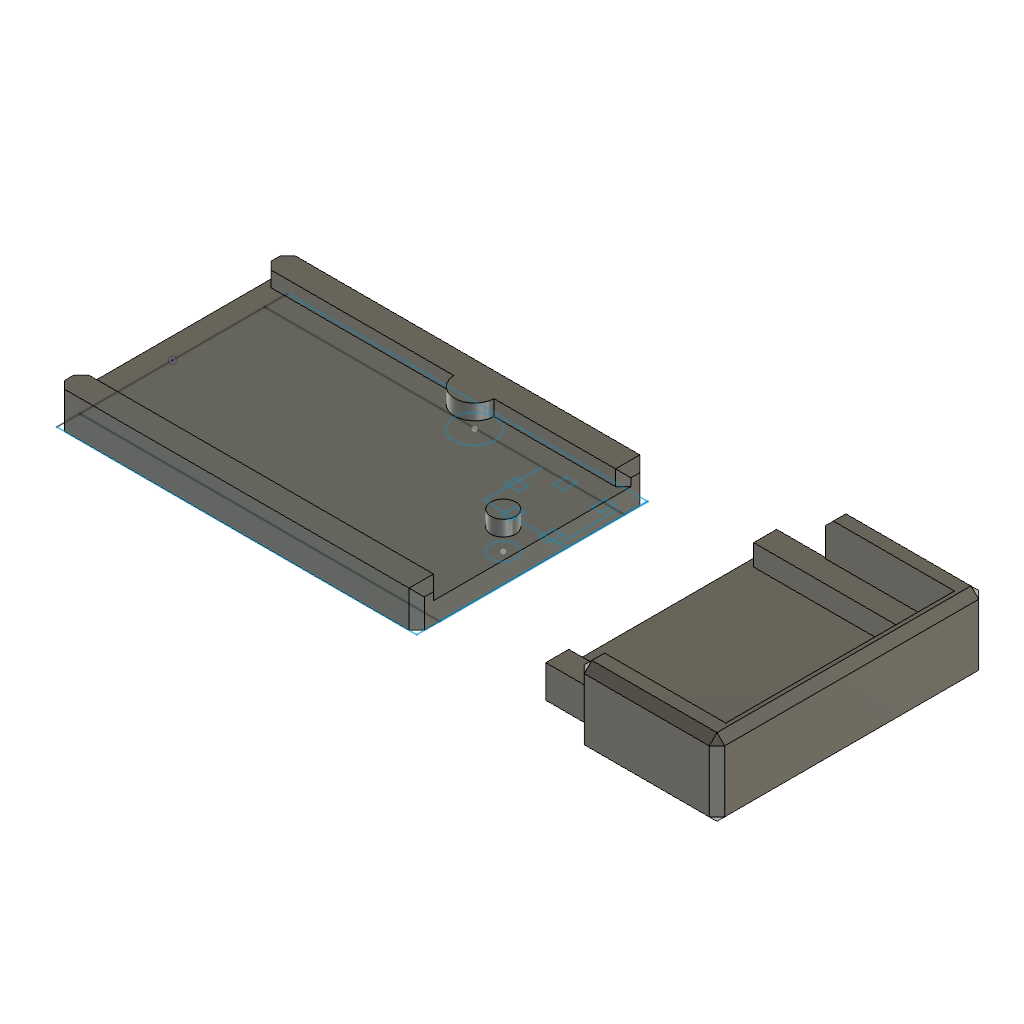
CH552_dongle (Autodesk Fusion 360 design; units mm, degrees)
description: Designed by EasyEDA Pro
part number: EasyEDA PCB Model~ES4X
Autodesk Fusion 360 part; units mm, degrees
sketch "スケッチ1" plane through (0, 0, 0) normal (0, 0, 1) x (1, 0, 0)
  line L0 (0, 4.8) -> (18.7, 4.8)
  line L1 (18.7, -4.8) -> (0, -4.8)
  line L2 (0, 4.8) -> (0, 6)
  line L3 (0, 6) -> (18.7, 6)
  line L4 (18.7, -6) -> (0, -6)
  line L5 (0, -6) -> (0, -4.8)
  circle A0 centre (17.195, 0) radius 0.65
  circle A1 centre (10.94, 4.77) radius 1.05
  line L6 (14.4, 4.8) -> (14.4, 1.8)
  line L7 (14.4, 1.8) -> (18.7, 1.8)
  line L8 (0, 0) -> (0, 4.8)
  line L9 (0, 0) -> (0, -4.8)
  line L10 (18.7, -4.8) -> (18.7, 6)
  line L11 (18.7, 6) -> (18.7, -6)
  line L12 (17.5, 5) -> (18, 5)
  line L13 (18, 5) -> (18, 4.3)
  line L14 (18, 4.3) -> (17.5, 4.3)
  line L15 (17.5, 4.3) -> (17.5, 5)
  line L16 (17.5, 2.3) -> (18, 2.3)
  line L17 (18, 2.3) -> (18, 1.6)
  line L18 (18, 1.6) -> (17.5, 1.6)
  line L19 (17.5, 1.6) -> (17.5, 2.3)
  line L20 (14.2, 3.6) -> (14.9, 3.6)
  line L21 (14.9, 3.6) -> (14.9, 3.1)
  line L22 (14.9, 3.1) -> (14.2, 3.1)
  line L23 (14.2, 3.1) -> (14.2, 3.6)
  line L24 (15.5, 5) -> (16, 5)
  line L25 (16, 5) -> (16, 4.3)
  line L26 (16, 4.3) -> (15.5, 4.3)
  line L27 (15.5, 4.3) -> (15.5, 5)
  line L28 (15.5, 2.3) -> (16, 2.3)
  line L29 (16, 2.3) -> (16, 1.6)
  line L30 (16, 1.6) -> (15.5, 1.6)
  line L31 (15.5, 1.6) -> (15.5, 2.3)
  line L32 (18.3, 4.8) -> (18.3, 1.8)
  dimension "d2" = 1.3
  dimension "d3" = 2.1
  dimension "d18" = 4.8
  dimension "d19" = 4.8
  dimension "d20" = 18.7
  constraint horizontal L0
  constraint horizontal L1
  constraint perpendicular L0 L2
  constraint perpendicular L1 L5
  constraint vertical L6
  constraint horizontal L7
  constraint coincident L0 L6.start
  constraint coincident L8.start L9.start
  constraint perpendicular L0 L8
  constraint perpendicular L1 L9
  constraint coincident L3 L10.end
  constraint perpendicular L3 L10
  constraint coincident L4 L11.end
  constraint coincident L0.end L10
  constraint coincident L0.end L11
  constraint coincident L7.end L10
  constraint horizontal L12
  constraint vertical L13
  constraint horizontal L14
  constraint vertical L15
  constraint horizontal L16
  constraint vertical L17
  constraint horizontal L18
  constraint vertical L19
  constraint horizontal L20
  constraint vertical L21
  constraint horizontal L22
  constraint vertical L23
  constraint horizontal L24
  constraint vertical L25
  constraint horizontal L26
  constraint vertical L27
  constraint horizontal L28
  constraint vertical L29
  constraint horizontal L30
  constraint vertical L31
  constraint coincident L0 L32.start
  constraint coincident L7 L32.end
  constraint perpendicular L7 L32
  measures "d2" diameter of A0
  measures "d3" diameter of A1
  measures "d18" distance of L0.start L8.start
  measures "d19" distance of L1.end L8.start
  measures "d20" distance of L1.start L1.end
extrude "押し出し1" add sketch "スケッチ1" along normal blind 1.1 contours L0 L6 L7 L13 L14 L15 L16 L17 L19 L20 L21 L22 L25 L26 L27 L28 L29 L31 L32 | L0 L7 L10 L11 L32 | L0 L13 L14 L15 | L0 L1 A1 L6 L7 L8 L9 L10 L11 L17 L18 L19 L20 L22 L23 L29 L30 L31 | L7 L17 L18 L19 | L7 L16 L17 L19 | L0 L25 L26 L27 | L7 L29 L30 L31 | L7 L28 L29 L31 | L6 L20 L21 L22 | L6 L20 L22 L23 makes body 1
extrude "押し出し2" add sketch "スケッチ1" along normal blind 1.9 contours L0 L2 L3 A1 L10 L11 L12 L13 L15 L24 L25 L27 | L0 L12 L13 L15 | L1 L4 L5 L11 | L0 L24 L25 L27 | L0 A1 | L0 A1 | A0 bodies 1
move_face "面をオフセット5" offset 0.07 3 faces at (6.2333, -4.8, 1.6333) (3.2968, 4.8, 1.3667) (14.2264, 4.8, 1.3667) on bodies 1
sketch "スケッチ2" plane through (0, 0, 0) normal (0, 0, 1) x (1, 0, 0)
  line L0 (25, 6) -> (25, 7)
  line L1 (25, 7) -> (35.3, 7)
  line L2 (35.3, 7) -> (35.3, -7)
  line L3 (35.3, -7) -> (25, -7)
  line L4 (25, -7) -> (25, -6)
  line L5 (25, 6) -> (25, -6)
  line L6 (25, 6) -> (34.7, 6)
  line L7 (34.7, -6) -> (25, -6)
  line L8 (34.7, -4.8) -> (25, -4.8)
  line L9 (34.7, 4.8) -> (25, 4.8)
  line L10 (28, 7) -> (28, -7)
  line L11 (34.7, -6) -> (34.7, 6)
  constraint vertical L0
  constraint perpendicular L0 L1
  constraint perpendicular L1 L2
  constraint perpendicular L2 L3
  constraint perpendicular L3 L4
  constraint parallel L4 L5
  constraint coincident L5 L8.end
  constraint coincident L5 L9.end
  constraint coincident L1 L10.start
  constraint coincident L3 L10.end
  constraint perpendicular L3 L10
  constraint coincident L9.start L11
  constraint perpendicular L9 L11
  constraint vertical L11
extrude "押し出し4" add sketch "スケッチ2" along normal blind 1 separate body contours L5 L8 L9 L10 | L8 L9 L10 L11 makes body 2
extrude "押し出し6" add sketch "スケッチ2" along normal blind 2.1 contours L5 L6 L9 L10 | L6 L9 L10 L11 | L5 L7 L8 L10 | L7 L8 L10 L11 bodies 2
extrude "押し出し5" add sketch "スケッチ2" along normal blind 4 contours L1 L2 L3 L6 L7 L10 L11 bodies 2
move_face "面をオフセット4" offset 0.06 2 faces at (30.2333, 6, 2.7333) (32.4667, -6, 2.7333) on bodies 2
chamfer "面取り6" distance 0.4 angle 45 23 edges at (28, 6.5, 0) (26.5, 6, 0) (25, 0, 0) (25, 6, 1.05) (25, -6, 1.05) (26.5, -6, 0) (28, -6.5, 0) (25, 4.8, 1.55) (25, -4.8, 1.55) (25, -5.4, 2.1) (25, 5.4, 2.1) (28, -6.47, 4) (28, 6.47, 4) (18.7, 4.73, 1.5) (18.7, 6, 0.95) (18.7, -4.73, 1.5) (18.7, -6, 0.95) (0, -6, 0.95) (0, -4.73, 1.5) (0, 4.73, 1.5) (0, 6, 0.95) (18.7, 5.365, 1.9) (18.7, -5.365, 1.9) 3 faces at (35.3, 2.3333, 1.3333) (32.8667, -7, 1.3333) (30.4333, 7, 1.3333) tangent chain off on bodies 1 2
named bodies: "shim", "cover"
